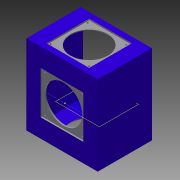
# Autodesk Inventor part: brain box bottom
Saved by Autodesk Inventor 2015 (Build 190159000, 159)
## iProperties
Created: 2014-09-09
Part Number: brain box bottom
Material: Generic
Document SubType Name: Modeling
Designer: ericd_000
Density: 1 g/cm^3
Appearance: Default
Author: ericd_000
Autodesk Inventor part; units mm, degrees
ref_plane "YZ Plane" through (0, 0, 0) normal (1, 0, 0) x (0, 1, 0)
ref_plane "XZ Plane" through (0, 0, 0) normal (0, 1, 0) x (-1, 0, 0)
ref_plane "XY Plane" through (0, 0, 0) normal (0, 0, 1) x (1, 0, 0)
sketch "Sketch1" plane through (0, 0, 0) normal (0, 1, 0) x (-1, 0, 0)
  line L0 (125, 140) -> (-125, 140)
  line L1 (-125, 140) -> (-125, -140)
  line L2 (-125, -140) -> (125, -140)
  line L3 (125, -140) -> (125, 140)
  point P0 (0, 0)
  point P1 (125, 0)
  point P2 (0, -140)
  dimension "d0" = 280
  dimension "d1" = 250
  constraints: 8 end point, 2 midpoint, 2 parallel, 1 horizontal, 1 horizontal alignment, 1 perpendicular, 1 vertical alignment
  measures "d0" distance of L2.end L0.start
  measures "d1" distance of L0.start L0.end
extrude "Extrusion1" add sketch "Sketch1" along normal blind 10
sketch "Sketch2" plane through (0, 10, 0) normal (0, 1, 0) x (1, 0, 0)
  line L0 (-125, -140) -> (125, -140)
  line L1 (125, -140) -> (125, 140)
  line L2 (125, 140) -> (-125, 140)
  line L3 (-125, 140) -> (-125, -140)
  line L4 (-117, -132) -> (117, -132)
  line L5 (117, -132) -> (117, 132)
  line L6 (117, 132) -> (-117, 132)
  line L7 (-117, 132) -> (-117, -132)
  point P0 (0, 0)
  dimension "d4" = 8
  constraints: 16 end point, 4 parallel, 2 perpendicular, 1 horizontal, 3 other
  measures "d4" distance between parallel lines of L3 L7
extrude "Extrusion2" add sketch "Sketch2" along normal blind 180
sketch "Sketch3" plane through (0, 190, 0) normal (0, 1, 0) x (1, 0, 0)
  circle A0 centre (-121, 136) radius 1.5
  circle A1 centre (121, 136) radius 1.5
  circle A2 centre (121, -136) radius 1.5
  circle A3 centre (-121, -136) radius 1.5
  line L0 (125, -140) -> (125, 140) projected
  line L1 (-125, -140) -> (125, -140) projected
  line L2 (125, 140) -> (-125, 140) projected
  line L3 (-125, 140) -> (-125, -140) projected
  point P0 (0, 0)
  dimension "d8" = 3
  dimension "d12" = 4
  dimension "d16" = 4
  dimension "d18" = 3
  dimension "d19" = 4
  dimension "d20" = 4
  dimension "d21" = 3
  dimension "d22" = 4
  dimension "d23" = 4
  dimension "d24" = 4
  dimension "d25" = 4
  dimension "d26" = 3
  constraints: 4 centre point
  measures "d8" diameter of A1
  measures "d12" distance from line of A1.centre L0
  measures "d16" distance from line of L2 A1.centre
  measures "d18" diameter of A0
  measures "d19" distance from line of L3 A0.centre
  measures "d20" distance from line of L2 A0.centre
  measures "d21" diameter of A2
  measures "d22" distance from line of L0 A2.centre
  measures "d23" distance from line of L1 A2.centre
  measures "d24" distance from line of L3 A3.centre
  measures "d25" distance from line of A3.centre L1
  measures "d26" diameter of A3
extrude "Extrusion3" cut sketch "Sketch3" against normal blind 15 contours A0 | A1 | A2 | A3
sketch "Sketch4" plane through (125, 0, 140) normal (1, 0, 0) x (0, 0, -1)
  line L0 (90, 145) -> (190, 145)
  line L1 (190, 145) -> (190, 45)
  line L2 (190, 45) -> (90, 45)
  line L3 (90, 45) -> (90, 145)
  line L4 (0, 190) -> (280, 190) projected
  line L5 (280, 0) -> (280, 190) projected
  point P0 (140, 0)
  point P1 (140, 145)
  point P2 (140, 190)
  point P3 (190, 95)
  point P4 (280, 95)
  dimension "d29" = 100
  dimension "d30" = 100
  constraints: 8 end point, 4 midpoint, 2 parallel, 1 horizontal, 1 horizontal alignment, 1 perpendicular, 1 vertical alignment
  measures "d29" distance of L0.start L0.end
  measures "d30" distance of L2.end L0.start
sketch "Sketch5" plane through (-125, 0, 140) normal (0, 0, 1) x (1, 0, 0)
  line L0 (250, 0) -> (250, 190) projected
  line L1 (0, 190) -> (250, 190) projected
  circle A0 centre (125, 95) radius 65.5
  point P0 (125, 0)
  point P1 (200.5, 95)
  point P2 (250, 95)
  point P3 (125, 163)
  point P4 (125, 190)
  point P5 (250, 95)
  point P6 (125, 190)
  dimension "d81" = 131
  constraints: 4 midpoint, 2 horizontal alignment, 2 vertical alignment, 1 centre point
  measures "d81" diameter of A0
extrude "Extrusion4" cut sketch "Sketch5" against normal blind 10
sketch "Sketch6" plane through (-125, 0, 140) normal (0, 0, 1) x (1, 0, 0)
  line L0 (200, 20) -> (50, 20)
  line L1 (50, 20) -> (50, 170)
  line L2 (50, 170) -> (200, 170)
  line L3 (200, 170) -> (200, 20)
  line L4 (0, 0) -> (250, 0) projected
  line L5 (0, 0) -> (0, 190) projected
  circle A0 centre (190, 30) radius 2.75
  circle A1 centre (190, 160) radius 2.75
  circle A2 centre (55, 30) radius 2.75
  circle A3 centre (55, 160) radius 2.75
  line L6 (195, 30) -> (55, 30)
  point P0 (125, 0)
  point P1 (49.5, 158)
  point P2 (180.5, 27)
  point P3 (125, 20)
  point P4 (125, 0)
  point P5 (50, 95)
  point P6 (0, 95)
  point P7 (60, 95)
  point P8 (125, 30)
  dimension "d108" = 150
  dimension "d109" = 150
  dimension "d112" = 5.5
  dimension "d113" = 10
  dimension "d114" = 10
  dimension "d117" = 130
  dimension "d120" = 135
  constraints: 10 end point, 5 midpoint, 4 centre point, 3 horizontal, 2 horizontal alignment, 2 parallel, 2 vertical alignment, 1 perpendicular, 1 vertical, 6 other
  measures "d108" distance of L0.start L0.end
  measures "d109" distance of L2.end L0.start
  measures "d112" diameter of A0
  measures "d113" distance from line of L3 A0.centre
  measures "d114" distance from line of L0 A0.centre
  measures "d117" distance of A0.centre A1.centre
  measures "d120" distance of A0.centre A2.centre
sketch "Sketch7" plane through (0, 10, 0) normal (0, 1, 0) x (1, 0, 0)
  line L0 (117, 132) -> (117, -132) construction
  line L1 (117, 0) -> (-117, 0) construction
  line L2 (-117, -132) -> (-117, 132) construction
  point P0 (0, 0)
  constraints: 3 midpoint, 2 end point
ref_plane "Work Plane1" through (117, 10, 0) normal (0, 0, -1) x (-1, 0, 0)
extrude "Extrusion13" cut sketch "Sketch6" against normal blind 5
mirror "Mirror2" about plane through (117, 10, 0) normal (0, 0, -1) of "Extrusion4"
sketch "Sketch8" plane through (0, 0, 0) normal (0, -1, 0) x (1, 0, 0)
  line L0 (75, -75) -> (-75, -75)
  line L1 (-75, -75) -> (-75, 75)
  line L2 (-75, 75) -> (75, 75)
  line L3 (75, 75) -> (75, -75)
  circle A0 centre (65, -65) radius 2.75
  circle A1 centre (65, 65) radius 2.75
  circle A2 centre (-65, -65) radius 2.75
  circle A3 centre (-65, 65) radius 2.75
  circle A4 centre (0, 0) radius 65.5
  point P0 (-35, 0)
  point P1 (0, -35)
  point P2 (75, 0)
  point P3 (0, -75)
  dimension "d58" = 130
  dimension "d65" = 130
  dimension "d82" = 131
  dimension "d83" = 150
  dimension "d84" = 150
  dimension "d85" = 10
  dimension "d86" = 10
  dimension "d87" = 130
  dimension "d88" = 130
  dimension "d89" = 5.5
  dimension "d90" = 5.5
  dimension "d91" = 5.5
  dimension "d92" = 5.5
  constraints: 8 end point, 5 centre point, 2 horizontal alignment, 2 midpoint, 2 parallel, 2 vertical alignment, 1 coincident, 1 perpendicular
  measures "d58" distance of A0.centre A1.centre
  measures "d65" distance of A0.centre A2.centre
  measures "d82" diameter of A4
  measures "d83" distance of L2.end L0.start
  measures "d84" distance of L0.start L0.end
  measures "d85" distance from line of L0 A0.centre
  measures "d86" distance from line of L1 A2.centre
  measures "d87" distance of A1.centre A3.centre
  measures "d88" distance of A2.centre A3.centre
  measures "d89" diameter of A0
  measures "d90" diameter of A2
  measures "d91" diameter of A3
  measures "d92" diameter of A1
extrude "Extrusion9" cut sketch "Sketch8" against normal blind 10 contours A4
sketch "Sketch13" plane through (0, 0, 0) normal (0, -1, 0) x (1, 0, 0)
  line L0 (-75, 75) -> (75, 75)
  line L1 (75, 75) -> (75, -75)
  line L2 (75, -75) -> (-75, -75)
  line L3 (-75, -75) -> (-75, 75)
  circle A0 centre (-65, 65) radius 2.75
  circle A1 centre (-65, -65) radius 2.75
  circle A2 centre (65, -65) radius 2.75
  circle A3 centre (65, 65) radius 2.75
  point P0 (0, 0)
  point P1 (75, 0)
  point P2 (0, 75)
  dimension "d95" = 150
  dimension "d96" = 150
  dimension "d97" = 5.5
  dimension "d98" = 10
  dimension "d99" = 10
  dimension "d102" = 360
  constraints: 8 end point, 4 centre point, 2 midpoint, 2 parallel, 1 horizontal, 1 horizontal alignment, 1 perpendicular, 1 vertical alignment, 9 other
  measures "d95" distance of L0.start L0.end
  measures "d96" distance of L2.end L0.start
  measures "d97" diameter of A0
  measures "d98" distance from line of L0 A0.centre
  measures "d99" distance from line of L3 A0.centre
extrude "Extrusion10" cut sketch "Sketch13" against normal blind 5
sketch "Sketch14" plane through (65, 0, 65) normal (0, -1, 0) x (1, 0, 0)
  circle A0 centre (0, 0) radius 2.75 projected
  circle A1 centre (0, 0) radius 2.75
  circle A2 centre (0, -130) radius 2.75 projected
  circle A3 centre (0, -130) radius 2.75
  circle A4 centre (-130, -130) radius 2.75 projected
  circle A5 centre (-130, -130) radius 2.75
  circle A6 centre (-130, 0) radius 2.75
  point P0 (-65, -65)
  constraints: 4 centre point, 3 coincident
extrude "Extrusion11" cut sketch "Sketch14" against normal up to next
sketch "Sketch16" plane through (-70, 160, 140) normal (0, 0, 1) x (1, 0, 0)
  circle A0 centre (0, 0) radius 2.75
  circle A1 centre (135, 0) radius 2.75
  circle A2 centre (135, 0) radius 2.75 projected
  circle A3 centre (135, -130) radius 2.75
  circle A4 centre (135, -130) radius 2.75 projected
  circle A5 centre (0, -130) radius 2.75
  circle A6 centre (0, -130) radius 2.75 projected
  circle A7 centre (0, 0) radius 2.75 projected
  point P0 (70, -160)
  dimension "d129" = 5.5
  dimension "d130" = 5.5
  dimension "d131" = 5.5
  dimension "d132" = 5.5
  constraints: 4 centre point, 4 concentric
  measures "d129" diameter of A1
  measures "d130" diameter of A3
  measures "d131" diameter of A5
  measures "d132" diameter of A0
extrude "Extrusion14" cut sketch "Sketch16" against normal blind 10
mirror "Mirror4" about plane through (117, 10, 0) normal (0, 0, -1) of "Extrusion13", "Extrusion14"
body "Solid1"
